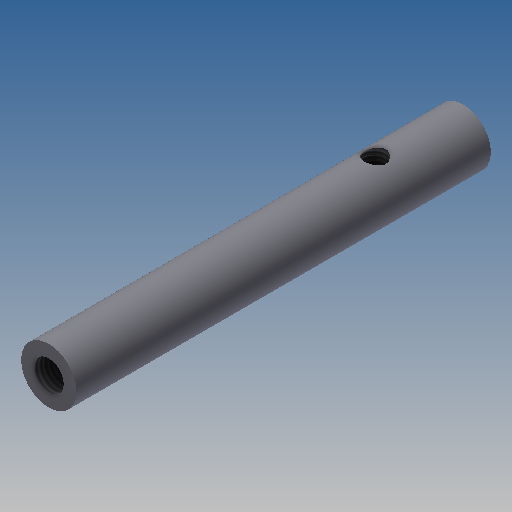
# Autodesk Inventor part: PWTR-0037
Saved by Autodesk Inventor 2021.1 (Build 251245000, 245)
## iProperties
Shininess: 64.0
Length Units: 11269
Angle Units: 11279
Time Units: 11290
Mass Units: 11284
Length Display Precision: 3
Angle Display Precision: 2
Compacted: True
Part Number: PWTR-0037
Document SubType Name: Modeling
Created: 2003-02-05
Designer: B. BOGAN
Material: Stainless Steel, 303
Description: Pitch Control Rod
Density: 7.75 g/cm^3
Mass: 84.3562 g
Surface Area: 46.7201 cm^2
Volume: 10.8847 cm^3
Appearance: Steel
Vendor: Non-Design Specific
Density: 0.0
Volumn: 0.0
Area: 0.0
PropertySet Name: Model Information
Control State: 0
Master: False
Checked Out: False
Title: PITCH CONTROL ROD
Author: B. BOGAN
Comments: Rev A: Length 3-1/2 was 3-3/8
Revision Number: B
Autodesk Inventor part; units mm, degrees
ref_plane "YZ Plane" through (0, 0, 0) normal (1, 0, 0) x (0, 1, 0)
ref_plane "XZ Plane" through (0, 0, 0) normal (0, 1, 0) x (-1, 0, 0)
sketch "Sketch1" plane through (0, 0, 0) normal (0, 0, 1) x (1, 0, 0)
  circle A0 centre (0, 0) radius 6.35
  dimension "d0" = 12.7
  constraints: 1 centre point
  measures "d0" diameter of A0
extrude "Extrusion1" add sketch "Sketch1" along normal blind 95.25
sketch "Sketch2" plane through (0, 0, 95.25) normal (0, 0, 1) x (1, 0, 0)
  circle A0 centre (0, 0) radius 6.35 projected
hole "Hole1" at (0, 0, 95.25) direction (0, 0, -1) diameter 6.9088 depth 19.05 tip angle 118 thread size "5/16-24 UNF" class "2B" standard "ANSI Unified Screw Threads"
ref_plane "Work Plane1" through (0, 6.35, 0) normal (0, 1, 0) x (-1, 0, 0)
sketch "Sketch3" plane through (0, 6.35, 0) normal (0, 1, 0) x (-1, 0, 0)
  line L0 (-6.35, 0) -> (6.35, 0) projected
  line L1 (-6.35, 95.25) -> (6.35, 95.25) projected
  line L2 (-6.35, 0) -> (6.35, 0) projected
  point P0 (0, 20.25)
  dimension "d18" = 75
  measures "d18" distance from line of point (0, 20.25) L1
hole "Hole2" at (0, 6.35, 20.25) direction (0, -1, 0) diameter 4.917 end through all thread size "M6x1" class "6H" standard "ISO Metric profile"
sketch "Sketch4" plane through (0, 0, 0) normal (0, 0, -1) x (-1, 0, 0)
  circle A0 centre (0, 0) radius 6.35 projected
hole "Hole3" at (0, 0, 0) direction (0, 0, 1) diameter 3.9624 depth 6.35 tip angle 118 thread size "10-32 UNF" class "2B" standard "ANSI Unified Screw Threads"
body "Solid1"
